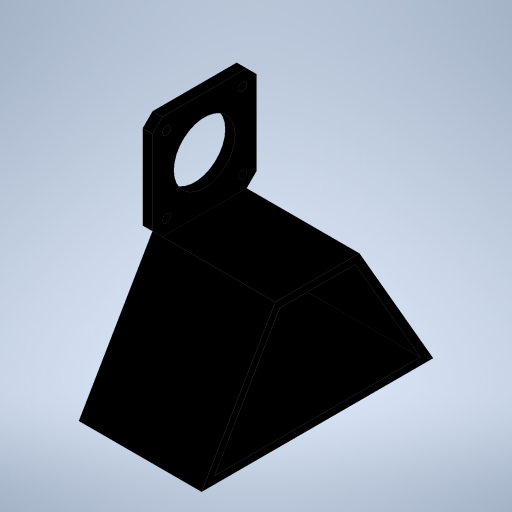
# Autodesk Inventor part: MotorHalterung
Saved by Autodesk Inventor 2023 (Build 270158000, 158)
## iProperties
Created: 2024-01-25
Part Number: MotorHalterung
Material: Generisch
Document SubType Name: Modeling
Designer: phili
Density: 1 g/cm^3
Appearance: Vorgabe
Author: phili
Autodesk Inventor part; units mm, degrees
ref_plane "YZ Plane" through (0, 0, 0) normal (1, 0, 0) x (0, 1, 0)
ref_plane "XZ Plane" through (0, 0, 0) normal (0, 1, 0) x (-1, 0, 0)
ref_plane "XY Plane" through (0, 0, 0) normal (0, 0, 1) x (1, 0, 0)
sketch "Skizze1" plane through (0, 0, 0) normal (1, 0, 0) x (0, 1, 0)
  line L0 (-21.15, -21.15) -> (21.15, -21.15)
  line L1 (21.15, -21.15) -> (21.15, 21.15)
  line L2 (21.15, 21.15) -> (-21.15, 21.15)
  line L3 (-21.15, 21.15) -> (-21.15, -21.15)
  line L4 (-21.15, -21.15) -> (21.15, 21.15) construction
  line L5 (21.15, -21.15) -> (-21.15, 21.15) construction
  point P0 (0, 0)
  dimension "d0" = 42.3
  dimension "d1" = 42.3
  constraints: 12 end point, 2 midpoint, 2 parallel, 1 horizontal, 1 perpendicular
  measures "d0" distance of L2.end L1.end
  measures "d1" distance of L1.end L0.end
extrude "Extrusion1" add sketch "Skizze1" along normal blind 4
chamfer "Fase1" distance 4 angle 45 4 edges at (2, 21.15, 21.15) (2, -21.15, 21.15) (2, -21.15, -21.15) (2, 21.15, -21.15)
sketch "Skizze2" plane through (4, 0, 0) normal (1, 0, 0) x (0, 0, -1)
  circle A0 centre (0, 0) radius 12.5
  dimension "d7" = 25
  constraints: 1 centre point, 1 coincident
  measures "d7" diameter of A0
extrude "Extrusion2" cut sketch "Skizze2" against normal blind 4
sketch "Skizze3" plane through (4, 0, 0) normal (1, 0, 0) x (0, 0, -1)
  point P0 (0, 0)
  point P1 (-15.5, 15.5)
  point P2 (15.5, 15.5)
  point P3 (15.5, -15.5)
  point P4 (-15.5, -15.5)
  dimension "d17" = 15.5
  dimension "d18" = 15.5
  dimension "d19" = 15.5
  dimension "d20" = 15.5
  dimension "d21" = 15.5
  dimension "d22" = 15.5
  dimension "d23" = 15.5
  dimension "d24" = 15.5
  measures "d17" horizontal distance of point (0, 0) point (-15.5, 15.5)
  measures "d18" horizontal distance of point (15.5, 15.5) point (0, 0)
  measures "d19" horizontal distance of point (0, 0) point (15.5, 15.5)
  measures "d20" horizontal distance of point (15.5, -15.5) point (0, 0)
  measures "d21" horizontal distance of point (15.5, -15.5) point (0, 0)
  measures "d22" horizontal distance of point (-15.5, -15.5) point (0, 0)
  measures "d23" horizontal distance of point (0, 0) point (-15.5, -15.5)
  measures "d24" horizontal distance of point (0, 0) point (-15.5, 15.5)
hole "Bohrung1" at (4, 15.5, 15.5) at (4, 15.5, -15.5) at (4, -15.5, -15.5) at (4, -15.5, 15.5) direction (-1, 0, 0) diameter 3.4 end through all
sketch "Skizze4" plane through (0, 0, 0) normal (-1, 0, 0) x (0, 0, 1)
  line L0 (17.15, -21.15) -> (-17.15, -21.15) projected
  line L1 (-17.15, -21.15) -> (-47.15, -73.1115)
  line L2 (-17.15, -21.15) -> (42.85, -21.15) construction
  line L3 (17.15, -21.15) -> (47.15, -73.1115)
  line L4 (17.15, -21.15) -> (77.15, -21.15) construction
  line L5 (-47.15, -73.1115) -> (47.15, -73.1115)
  line L6 (21.15, -17.15) -> (17.15, -21.15) projected
  line L7 (-17.15, -21.15) -> (17.15, -21.15)
  point P0 (0, 0)
  dimension "d25" = 60
  dimension "d27" = 60
  dimension "d28" = 60
  dimension "d29" = 60
  constraints: 12 end point, 3 horizontal, 2 equal length
  measures "d25" distance of L0.end L1.end
  measures "d27" distance of L0.start L3.end
  measures "d28" angle of L3 L4
  measures "d29" angle of L0 L1
extrude "Extrusion3" add sketch "Skizze4" against normal blind 50
shell "Wandung1" thickness 3 removed faces 1 at (50, -55.791, 5.7167)
sketch "Skizze8" plane through (0, 0, 0) normal (-1, 0, 0) x (0, 0, 1)
  line L0 (-15.4179, -24.15) -> (15.4179, -24.15) projected
  line L1 (-15.4179, -24.15) -> (15.4179, -24.15)
  line L2 (-41.9538, -70.1115) -> (41.9538, -70.1115) projected
  line L3 (15.4179, -24.15) -> (41.9538, -70.1115)
  line L4 (41.9538, -70.1115) -> (-41.9538, -70.1115)
  line L5 (-41.9538, -70.1115) -> (-15.4179, -24.15)
  point P0 (0, 0)
  constraints: 8 end point, 1 collinear, 1 parallel
extrude "Extrusion4" cut sketch "Skizze8" against normal blind 50
